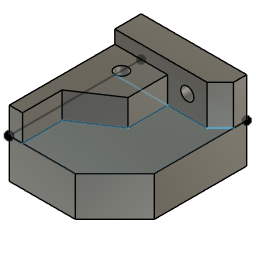
1 (Autodesk Fusion 360 design; units mm, degrees)
Autodesk Fusion 360 part; units mm, degrees
sketch "Sketch1" plane through (0, 0, 0) normal (0, 0, 1) x (1, 0, 0)
  line L0 (0, 0) -> (0, 200)
  line L1 (0, 200) -> (160, 200)
  line L2 (160, 200) -> (160, 60)
  line L3 (0, 0) -> (100, 0)
  line L4 (100, 0) -> (160, 60)
  constraint coincident L0.start L3.start
  constraint vertical L0
  constraint perpendicular L0 L1
  constraint perpendicular L1 L2
  constraint perpendicular L0 L3
extrude "Extrude1" add sketch "Sketch1" along normal blind 60
sketch "Sketch2" plane through (0, 0, 60) normal (0, 0, 1) x (-1, 0, 0)
  line L0 (0, 0) -> (-100, 0)
  line L1 (-100, 0) -> (-160, -60)
  line L2 (-160, -60) -> (-160, -200)
  line L3 (-160, -200) -> (0, -200)
  line L4 (0, -200) -> (0, 0)
  line L5 (0, 0) -> (0, -160)
  line L6 (0, -160) -> (-80, -160)
  line L7 (-80, -160) -> (-80, -100)
  line L8 (0, 0) -> (-20, 0)
  line L9 (-20, 0) -> (-20, -60)
  line L10 (-20, -60) -> (-80, -100)
  line L11 (0, -160) -> (0, -200)
  line L12 (-160, -200) -> (-160, -180)
  line L13 (-160, -180) -> (-140, -160)
  line L14 (-140, -160) -> (-80, -160)
  constraint coincident L0.start L4.end
  constraint perpendicular L0 L5
  constraint perpendicular L5 L6
  constraint perpendicular L6 L7
  constraint perpendicular L5 L8
  constraint perpendicular L8 L9
  constraint coincident L3.end L4.start
  constraint coincident L2.end L3.start
  constraint perpendicular L3 L12
  constraint perpendicular L7 L14
extrude "Extrude2" add sketch "Sketch2" along normal blind 40 contours L0 L4 L5 L6 L7 L8 L9 L10
extrude "Extrude3" add sketch "Sketch2" along normal blind 60 contours L2 L3 L4 L6 L11 L12 L13 L14
sketch "Sketch3" plane through (0, 160, 0) normal (0, -1, 0) x (1, 0, 0)
  line L0 (0, 100) -> (80, 100)
  line L1 (80, 100) -> (80, 60)
  line L2 (80, 60) -> (140, 60)
  line L3 (140, 60) -> (140, 120)
  line L4 (140, 120) -> (0, 120)
  line L5 (0, 120) -> (0, 100)
  circle A0 centre (110, 90) radius 10
  line L6 (110, 90) -> (110, 120)
  dimension "d17" = 20
  constraint coincident A0.centre L6.start
  constraint coincident L4 L6.end
  constraint perpendicular L4 L6
  measures "d17" diameter of A0
hole "Hole1" at (110, 160, 90) direction (0, 1, 0) diameter 20 depth 40 tip angle 118
sketch "Sketch4" plane through (0, 0, 100) normal (0, 0, 1) x (-1, 0, 0)
  line L0 (0, 0) -> (-20, 0)
  line L1 (-20, 0) -> (-20, -60)
  line L2 (-20, -60) -> (-80, -100)
  line L3 (-80, -100) -> (-80, -160)
  line L4 (-80, -160) -> (0, -160)
  line L5 (0, -160) -> (0, 0)
hole "Hole2" at (40, 130, 100) direction (0, 0, -1) diameter 20 depth 1000 tip angle 118
